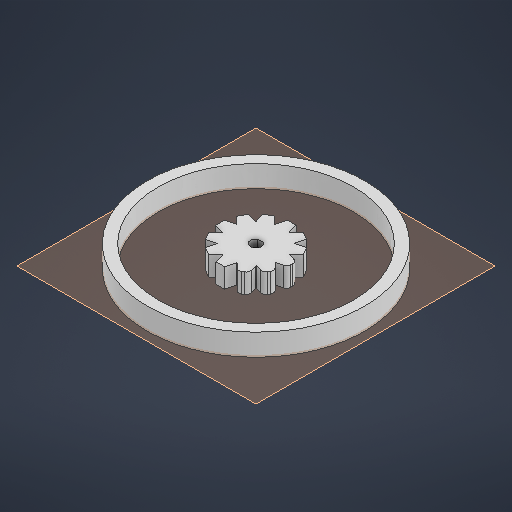
# Autodesk Inventor part: ringGEAR
Saved by Autodesk Inventor 2027.1 (Build 311267000, 267)
## iProperties
Created: 2026-10-02
Part Number: ringGEAR
Material: Generic
Document SubType Name: Modeling
Designer: HP
Density: 1 g/cm^3
Appearance: Default
Author: HP
Autodesk Inventor part; units mm, degrees
ref_plane "YZ Plane" through (0, 0, 0) normal (1, 0, 0) x (0, 1, 0)
ref_plane "XZ Plane" through (0, 0, 0) normal (0, 1, 0) x (-1, 0, 0)
ref_plane "XY Plane" through (0, 0, 0) normal (0, 0, 1) x (1, 0, 0)
sketch "Sketch1" plane through (0, 0, 0) normal (0, 1, 0) x (-1, 0, 0)
  circle A0 centre (0, 0) radius 45
  circle A1 centre (0, 0) radius 50
  dimension "d0" = 90
  dimension "d1" = 100
  constraints: 2 centre point, 2 coincident
  measures "d0" diameter of A0
  measures "d1" diameter of A1
extrude "Extrusion1" add sketch "Sketch1" along normal blind 10
ref_plane "Work Plane1" through (0, 1, 0) normal (0, 1, 0) x (1, 0, 0)
sketch "Sketch2" plane through (0, 1, 0) normal (0, 1, 0) x (1, 0, 0)
  circle A0 centre (0, 0) radius 12.5
  line L0 (-12.5, -0.0222) -> (-16.5, -0.0222)
  line L1 (-16.5, -0.0222) -> (-16.5, 1.9778)
  line L2 (-16.5, 1.9778) -> (-12.0944, 3.1583)
  line L3 (-16.5, -0.0222) -> (-16.5, -2.0222)
  line L4 (-16.5, -2.0222) -> (-12.0819, -3.206)
  arc A1 (-12.0944, 3.1583) -> (-12.0819, -3.206) centre (0, 0) ccw
  line L5 (-10.8142, -6.2692) -> (-14.2783, -8.2692)
  line L6 (-14.2783, -8.2692) -> (-15.2783, -6.5372)
  line L7 (-15.2783, -6.5372) -> (-12.0532, -3.3121)
  line L8 (-14.2783, -8.2692) -> (-13.2783, -10.0013)
  line L9 (-13.2783, -10.0013) -> (-8.8602, -8.8174)
  arc A2 (-12.0532, -3.3121) -> (-8.8602, -8.8174) centre (0, 0) ccw
  line L10 (-6.2308, -10.8364) -> (-8.2308, -14.3005)
  line L11 (-8.2308, -14.3005) -> (-9.9628, -13.3005)
  line L12 (-9.9628, -13.3005) -> (-8.7823, -8.895)
  line L13 (-8.2308, -14.3005) -> (-6.4987, -15.3005)
  line L14 (-6.4987, -15.3005) -> (-3.2644, -12.0662)
  arc A3 (-8.7823, -8.895) -> (-3.2644, -12.0662) centre (0, 0) ccw
  line L15 (0.0222, -12.5) -> (0.0222, -16.5)
  line L16 (0.0222, -16.5) -> (-1.9778, -16.5)
  line L17 (-1.9778, -16.5) -> (-3.1583, -12.0944)
  line L18 (0.0222, -16.5) -> (2.0222, -16.5)
  line L19 (2.0222, -16.5) -> (3.206, -12.0819)
  arc A4 (-3.1583, -12.0944) -> (3.206, -12.0819) centre (0, 0) ccw
  line L20 (6.2692, -10.8142) -> (8.2692, -14.2783)
  line L21 (8.2692, -14.2783) -> (6.5372, -15.2783)
  line L22 (6.5372, -15.2783) -> (3.3121, -12.0532)
  line L23 (8.2692, -14.2783) -> (10.0013, -13.2783)
  line L24 (10.0013, -13.2783) -> (8.8174, -8.8602)
  arc A5 (3.3121, -12.0532) -> (8.8174, -8.8602) centre (0, 0) ccw
  line L25 (10.8364, -6.2308) -> (14.3005, -8.2308)
  line L26 (14.3005, -8.2308) -> (13.3005, -9.9628)
  line L27 (13.3005, -9.9628) -> (8.895, -8.7823)
  line L28 (14.3005, -8.2308) -> (15.3005, -6.4987)
  line L29 (15.3005, -6.4987) -> (12.0662, -3.2644)
  arc A6 (8.895, -8.7823) -> (12.0662, -3.2644) centre (0, 0) ccw
  line L30 (12.5, 0.0222) -> (16.5, 0.0222)
  line L31 (16.5, 0.0222) -> (16.5, -1.9778)
  line L32 (16.5, -1.9778) -> (12.0944, -3.1583)
  line L33 (16.5, 0.0222) -> (16.5, 2.0222)
  line L34 (16.5, 2.0222) -> (12.0819, 3.206)
  arc A7 (12.0944, -3.1583) -> (12.0819, 3.206) centre (0, 0) ccw
  line L35 (10.8142, 6.2692) -> (14.2783, 8.2692)
  line L36 (14.2783, 8.2692) -> (15.2783, 6.5372)
  line L37 (15.2783, 6.5372) -> (12.0532, 3.3121)
  line L38 (14.2783, 8.2692) -> (13.2783, 10.0013)
  line L39 (13.2783, 10.0013) -> (8.8602, 8.8174)
  arc A8 (12.0532, 3.3121) -> (8.8602, 8.8174) centre (0, 0) ccw
  line L40 (6.2308, 10.8364) -> (8.2308, 14.3005)
  line L41 (8.2308, 14.3005) -> (9.9628, 13.3005)
  line L42 (9.9628, 13.3005) -> (8.7823, 8.895)
  line L43 (8.2308, 14.3005) -> (6.4987, 15.3005)
  line L44 (6.4987, 15.3005) -> (3.2644, 12.0662)
  arc A9 (8.7823, 8.895) -> (3.2644, 12.0662) centre (0, 0) ccw
  line L45 (-0.0222, 12.5) -> (-0.0222, 16.5)
  line L46 (-0.0222, 16.5) -> (1.9778, 16.5)
  line L47 (1.9778, 16.5) -> (3.1583, 12.0944)
  line L48 (-0.0222, 16.5) -> (-2.0222, 16.5)
  line L49 (-2.0222, 16.5) -> (-3.206, 12.0819)
  arc A10 (3.1583, 12.0944) -> (-3.206, 12.0819) centre (0, 0) ccw
  line L50 (-6.2692, 10.8142) -> (-8.2692, 14.2783)
  line L51 (-8.2692, 14.2783) -> (-6.5372, 15.2783)
  line L52 (-6.5372, 15.2783) -> (-3.3121, 12.0532)
  line L53 (-8.2692, 14.2783) -> (-10.0013, 13.2783)
  line L54 (-10.0013, 13.2783) -> (-8.8174, 8.8602)
  arc A11 (-3.3121, 12.0532) -> (-8.8174, 8.8602) centre (0, 0) ccw
  line L55 (-10.8364, 6.2308) -> (-14.3005, 8.2308)
  line L56 (-14.3005, 8.2308) -> (-13.3005, 9.9628)
  line L57 (-13.3005, 9.9628) -> (-8.895, 8.7823)
  line L58 (-14.3005, 8.2308) -> (-15.3005, 6.4987)
  line L59 (-15.3005, 6.4987) -> (-12.0662, 3.2644)
  arc A12 (-8.895, 8.7823) -> (-12.0662, 3.2644) centre (0, 0) ccw
  circle A13 centre (0, 0) radius 2.5527
  line L60 (-1.4351, 2.1111) -> (1.4351, 2.1111)
  dimension "d5" = 25
  dimension "d6" = 105
  dimension "d7" = 105
  dimension "d8" = 2
  dimension "d9" = 2
  dimension "d10" = 4
  dimension "d13" = 360
  dimension "d17" = 5.1054
  dimension "d18" = 2.8702
  constraints: 122 end point, 38 point on circle, 13 centre point, 12 point on line, 2 coincident, 2 horizontal, 1 perpendicular, 162 other
  measures "d6" angle of L3 L4
  measures "d7" angle of L2 L1
  measures "d8" distance of L0.end L3.end
  measures "d9" distance of L0.end L1.end
  measures "d10" distance of L0.start L0.end
  measures "d17" diameter of A13
  measures "d18" distance of L60.start L60.end
extrude "Extrusion2" add sketch "Sketch2" along normal blind 9 contours A0 | A0 L30 L31 L32 | A0 L34 L33 L30 | L29 L28 L25 A0 | A0 L35 L36 L37 | L25 L26 L27 A0 | A0 L39 L38 L35 | L24 L23 L20 A0 | A0 L40 L41 L42 | L20 L21 L22 A0 | A0 L44 L43 L40 | L19 L18 L15 A0 | A0 L45 L46 L47 | L15 L16 L17 A0 | A0 L49 L48 L45 | L14 L13 L10 A0 | A0 L50 L51 L52 | L10 L11 L12 A0 | A0 L54 L53 L50 | L9 L8 L5 A0 | A0 L55 L56 L57 | L5 L6 L7 A0 | A0 L59 L58 L55 | L4 L3 L0 A0 | A0 L0 L1 L2 | L60 A13 picked at (-0.1014, 2.2522)
fillet "Fillet3" radius 2 2 edges at (16.5, 5.5, 1.9778) (16.5, 5.5, -2.0222)
fillet "Fillet4" radius 2 4 edges at (13.3005, 5.5, 9.9628) (15.3005, 5.5, 6.4987) (10.0013, 5.5, 13.2783) (6.5372, 5.5, 15.2783)
equation "\"d8\" = d9"
body "Solid1"
